Autodesk Fusion 360 part; units mm, degrees
(part 2 of 3)
pattern_linear "R-Pattern3" count 15 spacing 2.54 along (1, 0, 0) count 25 spacing 2.5396 along (0, 0, -1) of bodies 3 2 4 makes body 5 at (3.4863, 1, 63.5089) makes body 6 at (6.5468, 1, 62.4281) makes body 7 at (9.0868, 1, 63.5219) makes body 8 at (11.6268, 1, 63.5219) makes body 9 at (14.1668, 1, 63.5219) makes body 10 at (16.7068, 1, 63.5219) makes body 11 at (19.2468, 1, 63.5219) makes body 12 at (21.7868, 1, 63.5219) makes body 13 at (24.3268, 1, 63.5219) makes body 14 at (26.8668, 1, 63.5219) makes body 15 at (29.4068, 1, 63.5219) makes body 16 at (32.2529, 1, 63.2081) makes body 17 at (34.4868, 1, 63.5219) makes body 18 at (37.0268, 1, 63.5219) makes body 19 at (4.654, 0, 62.8955) makes body 20 at (7.194, 0, 62.8955) makes body 21 at (9.7359, 0, 62.9204) makes body 22 at (12.2759, 0, 62.9204) makes body 23 at (14.8159, 0, 62.9204) makes body 24 at (17.354, 0, 62.8955) makes body 25 at (19.894, 0, 62.8955) makes body 26 at (22.434, 0, 62.8955) makes body 27 at (24.974, 0, 62.8955) makes body 28 at (27.514, 0, 62.8955) makes body 29 at (30.054, 0, 62.8955) makes body 30 at (32.594, 0, 62.8955) makes body 31 at (35.134, 0, 62.8955) makes body 32 at (37.674, 0, 62.8955) makes body 33 at (4.654, 1.5, 62.8955) makes body 34 at (7.194, 1.5, 62.8955) makes body 35 at (9.7359, 1.5, 62.9204) makes body 36 at (12.2759, 1.5, 62.9204) makes body 37 at (14.8159, 1.5, 62.9204) makes body 38 at (17.354, 1.5, 62.8955) makes body 39 at (19.894, 1.5, 62.8955) makes body 40 at (22.434, 1.5, 62.8955) makes body 41 at (24.974, 1.5, 62.8955) makes body 42 at (27.514, 1.5, 62.8955) makes body 43 at (30.054, 1.5, 62.8955) makes body 44 at (32.594, 1.5, 62.8955) makes body 45 at (35.134, 1.5, 62.8955) makes body 46 at (37.674, 1.5, 62.8955) makes body 47 at (1.4668, 1, 60.9823) makes body 48 at (3.4863, 1, 60.9693) makes body 49 at (6.5468, 1, 59.8885) makes body 50 at (9.0868, 1, 60.9823) makes body 51 at (11.6268, 1, 60.9823) makes body 52 at (14.1668, 1, 60.9823) makes body 53 at (16.7068, 1, 60.9823) makes body 54 at (19.2468, 1, 60.9823) makes body 55 at (21.7868, 1, 60.9823) makes body 56 at (24.3268, 1, 60.9823) makes body 57 at (26.8668, 1, 60.9823) makes body 58 at (29.4068, 1, 60.9823) makes body 59 at (32.2529, 1, 60.6685) makes body 60 at (34.4868, 1, 60.9823) makes body 61 at (37.0268, 1, 60.9823) makes body 62 at (1.4668, 1, 58.4427) makes body 63 at (3.4863, 1, 58.4298) makes body 64 at (6.5468, 1, 57.3489) makes body 65 at (9.0868, 1, 58.4427) makes body 66 at (11.6268, 1, 58.4427) makes body 67 at (14.1668, 1, 58.4427) makes body 68 at (16.7068, 1, 58.4427) makes body 69 at (19.2468, 1, 58.4427) makes body 70 at (21.7868, 1, 58.4427) makes body 71 at (24.3268, 1, 58.4427) makes body 72 at (26.8668, 1, 58.4427) makes body 73 at (29.4068, 1, 58.4427) makes body 74 at (32.2529, 1, 58.1289) makes body 75 at (34.4868, 1, 58.4427) makes body 76 at (37.0268, 1, 58.4427) makes body 77 at (1.4668, 1, 55.9032) makes body 78 at (3.4863, 1, 55.8902) makes body 79 at (6.5468, 1, 54.8093) makes body 80 at (9.0868, 1, 55.9032) makes body 81 at (11.6268, 1, 55.9032) makes body 82 at (14.1668, 1, 55.9032) makes body 83 at (16.7068, 1, 55.9032) makes body 84 at (19.2468, 1, 55.9032) makes body 85 at (21.7868, 1, 55.9032) makes body 86 at (24.3268, 1, 55.9032) makes body 87 at (26.8668, 1, 55.9032) makes body 88 at (29.4068, 1, 55.9032) makes body 89 at (32.2529, 1, 55.5893) makes body 90 at (34.4868, 1, 55.9032) makes body 91 at (37.0268, 1, 55.9032) makes body 92 at (1.4668, 1, 53.3636) makes body 93 at (3.4863, 1, 53.3506) makes body 94 at (6.5468, 1, 52.2698) makes body 95 at (9.0868, 1, 53.3636) makes body 96 at (11.6268, 1, 53.3636) makes body 97 at (14.1668, 1, 53.3636) makes body 98 at (16.7068, 1, 53.3636) makes body 99 at (19.2468, 1, 53.3636) makes body 100 at (21.7868, 1, 53.3636) makes body 101 at (24.3268, 1, 53.3636) makes body 102 at (26.8668, 1, 53.3636) makes body 103 at (29.4068, 1, 53.3636) makes body 104 at (32.2529, 1, 53.0497) makes body 105 at (34.4868, 1, 53.3636) makes body 106 at (37.0268, 1, 53.3636) makes body 107 at (1.4668, 1, 50.824) makes body 108 at (3.4863, 1, 50.811) makes body 109 at (6.5468, 1, 49.7302) makes body 110 at (9.0868, 1, 50.824) makes body 111 at (11.6268, 1, 50.824) makes body 112 at (14.1668, 1, 50.824) makes body 113 at (16.7068, 1, 50.824) makes body 114 at (19.2468, 1, 50.824) makes body 115 at (21.7868, 1, 50.824) makes body 116 at (24.3268, 1, 50.824) makes body 117 at (26.8668, 1, 50.824) makes body 118 at (29.4068, 1, 50.824) makes body 119 at (32.2529, 1, 50.5101) makes body 120 at (34.4868, 1, 50.824) makes body 121 at (37.0268, 1, 50.824) makes body 122 at (1.4668, 1, 48.2844) makes body 123 at (3.4863, 1, 48.2714) makes body 124 at (6.5468, 1, 47.1906) makes body 125 at (9.0868, 1, 48.2844) makes body 126 at (11.6268, 1, 48.2844) makes body 127 at (14.1668, 1, 48.2844) makes body 128 at (16.7068, 1, 48.2844) makes body 129 at (19.2468, 1, 48.2844) makes body 130 at (21.7868, 1, 48.2844) makes body 131 at (24.3268, 1, 48.2844) makes body 132 at (26.8668, 1, 48.2844) makes body 133 at (29.4068, 1, 48.2844) makes body 134 at (32.2529, 1, 47.9706) makes body 135 at (34.4868, 1, 48.2844) makes body 136 at (37.0268, 1, 48.2844) makes body 137 at (1.4668, 1, 45.7448) makes body 138 at (3.4863, 1, 45.7318) makes body 139 at (6.5468, 1, 44.651) makes body 140 at (9.0868, 1, 45.7448) makes body 141 at (11.6268, 1, 45.7448) makes body 142 at (14.1668, 1, 45.7448) makes body 143 at (16.7068, 1, 45.7448) makes body 144 at (19.2468, 1, 45.7448) makes body 145 at (21.7868, 1, 45.7448) makes body 146 at (24.3268, 1, 45.7448) makes body 147 at (26.8668, 1, 45.7448) makes body 148 at (29.4068, 1, 45.7448) makes body 149 at (32.2529, 1, 45.431) makes body 150 at (34.4868, 1, 45.7448) makes body 151 at (37.0268, 1, 45.7448) makes body 152 at (1.4668, 1, 43.2052) makes body 153 at (3.4863, 1, 43.1923) makes body 154 at (6.5468, 1, 42.1114) makes body 155 at (9.0868, 1, 43.2052) makes body 156 at (11.6268, 1, 43.2052) makes body 157 at (14.1668, 1, 43.2052) makes body 158 at (16.7068, 1, 43.2052) makes body 159 at (19.2468, 1, 43.2052) makes body 160 at (21.7868, 1, 43.2052) makes body 161 at (24.3268, 1, 43.2052) makes body 162 at (26.8668, 1, 43.2052) makes body 163 at (29.4068, 1, 43.2052) makes body 164 at (32.2529, 1, 42.8914) makes body 165 at (34.4868, 1, 43.2052) makes body 166 at (37.0268, 1, 43.2052) makes body 167 at (1.4668, 1, 40.6657) makes body 168 at (3.4863, 1, 40.6527) makes body 169 at (6.5468, 1, 39.5718) makes body 170 at (9.0868, 1, 40.6657) makes body 171 at (11.6268, 1, 40.6657) makes body 172 at (14.1668, 1, 40.6657) makes body 173 at (16.7068, 1, 40.6657) makes body 174 at (19.2468, 1, 40.6657) makes body 175 at (21.7868, 1, 40.6657) makes body 176 at (24.3268, 1, 40.6657) makes body 177 at (26.8668, 1, 40.6657) makes body 178 at (29.4068, 1, 40.6657) makes body 179 at (32.2529, 1, 40.3518) makes body 180 at (34.4868, 1, 40.6657) makes body 181 at (37.0268, 1, 40.6657) makes body 182 at (1.4668, 1, 38.1261) makes body 183 at (3.4863, 1, 38.1131) makes body 184 at (6.5468, 1, 37.0323) makes body 185 at (9.0868, 1, 38.1261) makes body 186 at (11.6268, 1, 38.1261) makes body 187 at (14.1668, 1, 38.1261) makes body 188 at (16.7068, 1, 38.1261) makes body 189 at (19.2468, 1, 38.1261) makes body 190 at (21.7868, 1, 38.1261) makes body 191 at (24.3268, 1, 38.1261) makes body 192 at (26.8668, 1, 38.1261) makes body 193 at (29.4068, 1, 38.1261) makes body 194 at (32.2529, 1, 37.8122) makes body 195 at (34.4868, 1, 38.1261) makes body 196 at (37.0268, 1, 38.1261) makes body 197 at (1.4668, 1, 35.5865) makes body 198 at (3.4863, 1, 35.5735) makes body 199 at (6.5468, 1, 34.4927) makes body 200 at (9.0868, 1, 35.5865) makes body 201 at (11.6268, 1, 35.5865) makes body 202 at (14.1668, 1, 35.5865) makes body 203 at (16.7068, 1, 35.5865) makes body 204 at (19.2468, 1, 35.5865) makes body 205 at (21.7868, 1, 35.5865) makes body 206 at (24.3268, 1, 35.5865) makes body 207 at (26.8668, 1, 35.5865) makes body 208 at (29.4068, 1, 35.5865) makes body 209 at (32.2529, 1, 35.2726) makes body 210 at (34.4868, 1, 35.5865) makes body 211 at (37.0268, 1, 35.5865) makes body 212 at (1.4668, 1, 33.0469) makes body 213 at (3.4863, 1, 33.0339) makes body 214 at (6.8993, 0.5, 32.5299) makes body 215 at (9.0868, 1, 33.0469) makes body 216 at (11.6268, 1, 33.0469) makes body 217 at (14.1668, 1, 33.0469) makes body 218 at (16.7068, 1, 33.0469) makes body 219 at (19.2468, 1, 33.0469) makes body 220 at (21.7868, 1, 33.0469) makes body 221 at (24.3268, 1, 33.0469) makes body 222 at (26.8668, 1, 33.0469) makes body 223 at (29.4068, 1, 33.0469) makes body 224 at (32.2529, 1, 32.7331) makes body 225 at (34.4868, 1, 33.0469) makes body 226 at (37.0268, 1, 33.0469) makes body 227 at (1.8193, 1, 29.9305) makes body 228 at (4.3593, 1, 29.9305) makes body 229 at (6.8993, 1, 29.9305) makes body 230 at (9.4393, 1, 29.9305) makes body 231 at (11.9793, 1, 29.9305) makes body 232 at (14.5193, 1, 29.9305) makes body 233 at (17.0593, 1, 29.9305) makes body 234 at (19.5993, 1, 29.9305) makes body 235 at (22.1393, 1, 29.9305) makes body 236 at (24.6793, 1, 29.9305) makes body 237 at (27.2193, 1, 29.9305) makes body 238 at (29.7593, 1, 29.9305) makes body 239 at (32.2993, 1, 29.9305) makes body 240 at (34.5902, 1, 30.4476) makes body 241 at (37.1302, 1, 30.4476) makes body 242 at (1.8193, 1, 27.3909) makes body 243 at (4.3593, 1, 27.3909) makes body 244 at (6.8993, 1, 27.3909) makes body 245 at (9.4393, 1, 27.3909) makes body 246 at (11.9793, 1, 27.3909) makes body 247 at (14.5193, 1, 27.3909) makes body 248 at (17.0593, 1, 27.3909) makes body 249 at (19.5993, 1, 27.3909) makes body 250 at (22.1393, 1, 27.3909) makes body 251 at (24.6793, 1, 27.3909) makes body 252 at (27.2193, 1, 27.3909) makes body 253 at (29.7593, 1, 27.3909) makes body 254 at (32.2993, 1, 27.3909) makes body 255 at (34.5902, 1, 27.908) makes body 256 at (37.1302, 1, 27.908) makes body 257 at (1.8193, 1, 24.8513) makes body 258 at (4.3593, 1, 24.8513) makes body 259 at (6.8993, 1, 24.8513) makes body 260 at (9.4393, 1, 24.8513) makes body 261 at (11.9793, 1, 24.8513) makes body 262 at (14.5193, 1, 24.8513) makes body 263 at (17.0593, 1, 24.8513) makes body 264 at (19.5993, 1, 24.8513) makes body 265 at (22.1393, 1, 24.8513) makes body 266 at (24.6793, 1, 24.8513) makes body 267 at (27.2193, 1, 24.8513) makes body 268 at (29.7593, 1, 24.8513) makes body 269 at (32.2993, 1, 24.8513) makes body 270 at (34.5902, 1, 25.3684) makes body 271 at (37.1302, 1, 25.3684) makes body 272 at (1.8193, 1, 22.3118) makes body 273 at (4.3593, 1, 22.3118) makes body 274 at (6.8993, 1, 22.3118) makes body 275 at (9.4393, 1, 22.3118) makes body 276 at (11.9793, 1, 22.3118) makes body 277 at (14.5193, 1, 22.3118) makes body 278 at (17.0593, 1, 22.3118) makes body 279 at (19.5993, 1, 22.3118) makes body 280 at (22.1393, 1, 22.3118) makes body 281 at (24.6793, 1, 22.3118) makes body 282 at (27.2193, 1, 22.3118) makes body 283 at (29.7593, 1, 22.3118) makes body 284 at (32.2993, 1, 22.3118) makes body 285 at (34.5902, 1, 22.8288) makes body 286 at (37.1302, 1, 22.8288) makes body 287 at (1.8193, 1, 19.7722) makes body 288 at (4.3593, 1, 19.7722) makes body 289 at (6.8993, 1, 19.7722) makes body 290 at (9.4393, 1, 19.7722) makes body 291 at (11.9793, 1, 19.7722) makes body 292 at (14.5193, 1, 19.7722) makes body 293 at (17.0593, 1, 19.7722) makes body 294 at (19.5993, 1, 19.7722) makes body 295 at (22.1393, 1, 19.7722) makes body 296 at (24.6793, 1, 19.7722) makes body 297 at (27.2193, 1, 19.7722) makes body 298 at (29.7593, 1, 19.7722) makes body 299 at (32.2993, 1, 19.7722) makes body 300 at (34.5902, 1, 20.2892) makes body 301 at (37.1302, 1, 20.2892) makes body 302 at (1.8193, 1, 17.2326) makes body 303 at (4.3593, 1, 17.2326) makes body 304 at (6.8993, 1, 17.2326) makes body 305 at (9.4393, 1, 17.2326) makes body 306 at (11.9793, 1, 17.2326) makes body 307 at (14.5193, 1, 17.2326) makes body 308 at (17.0593, 1, 17.2326) makes body 309 at (19.5993, 1, 17.2326) makes body 310 at (22.1393, 1, 17.2326) makes body 311 at (24.6793, 1, 17.2326) makes body 312 at (27.2193, 1, 17.2326) makes body 313 at (29.7593, 1, 17.2326) makes body 314 at (32.2993, 1, 17.2326) makes body 315 at (34.5902, 1, 17.7497) makes body 316 at (37.1302, 1, 17.7497) makes body 317 at (0.7604, 1, 14.3372) makes body 318 at (4.157, 1, 15.1728) makes body 319 at (6.697, 1, 15.1728) makes body 320 at (9.237, 1, 15.1728) makes body 321 at (11.777, 1, 15.1728) makes body 322 at (14.317, 1, 15.1728) makes body 323 at (16.972, 1, 15.0358) makes body 324 at (19.512, 1, 15.0358) makes body 325 at (22.052, 1, 15.0358) makes body 326 at (24.592, 1, 15.0358) makes body 327 at (27.132, 1, 15.0358) makes body 328 at (29.672, 1, 15.0358) makes body 329 at (31.1731, 1, 15.0099) makes body 330 at (34.5902, 1, 15.2101) makes body 331 at (37.1302, 1, 15.2101) makes body 332 at (0.7604, 1, 11.7977) makes body 333 at (4.157, 1, 12.6332) makes body 334 at (6.697, 1, 12.6332) makes body 335 at (9.237, 1, 12.6332) makes body 336 at (11.777, 1, 12.6332) makes body 337 at (14.317, 1, 12.6332) makes body 338 at (16.972, 1, 12.4962) makes body 339 at (19.512, 1, 12.4962) makes body 340 at (22.052, 1, 12.4962) makes body 341 at (24.592, 1, 12.4962) makes body 342 at (27.132, 1, 12.4962) makes body 343 at (29.672, 1, 12.4962) makes body 344 at (31.1731, 1, 12.4703) makes body 345 at (34.5902, 1, 12.6705) makes body 346 at (37.1302, 1, 12.6705) makes body 347 at (0.7604, 1, 9.2581) makes body 348 at (4.157, 1, 10.0936) makes body 349 at (6.697, 1, 10.0936) makes body 350 at (9.237, 1, 10.0936) makes body 351 at (11.777, 1, 10.0936) makes body 352 at (14.317, 1, 10.0936) makes body 353 at (16.972, 1, 9.9566) makes body 354 at (19.512, 1, 9.9566) makes body 355 at (22.052, 1, 9.9566) makes body 356 at (24.592, 1, 9.9566) makes body 357 at (27.132, 1, 9.9566) makes body 358 at (29.672, 1, 9.9566) makes body 359 at (31.1731, 1, 9.9307) makes body 360 at (34.5902, 1, 10.1309) makes body 361 at (37.1302, 1, 10.1309) makes body 362 at (1.8193, 1, 7.0743) makes body 363 at (4.3593, 1, 7.0743) makes body 364 at (6.8993, 1, 7.0743) makes body 365 at (9.4393, 1, 7.0743) makes body 366 at (11.9793, 1, 7.0743) makes body 367 at (14.5193, 1, 7.0743) makes body 368 at (17.0593, 1, 7.0743) makes body 369 at (19.5993, 1, 7.0743) makes body 370 at (22.1393, 1, 7.0743) makes body 371 at (24.6793, 1, 7.0743) makes body 372 at (27.2193, 1, 7.0743) makes body 373 at (29.7593, 1, 7.0743) makes body 374 at (32.2529, 1, 7.3372) makes body 375 at (34.5902, 1, 7.5913) makes body 376 at (37.1302, 1, 7.5913) makes body 377 at (1.8193, 1, 4.5347) makes body 378 at (4.3593, 1, 4.5347) makes body 379 at (6.8993, 1, 4.5347) makes body 380 at (9.4393, 1, 4.5347) makes body 381 at (11.9793, 1, 4.5347) makes body 382 at (14.5193, 1, 4.5347) makes body 383 at (17.0593, 1, 4.5347) makes body 384 at (19.5993, 1, 4.5347) makes body 385 at (22.1393, 1, 4.5347) makes body 386 at (24.6793, 1, 4.5347) makes body 387 at (27.2193, 1, 4.5347) makes body 388 at (29.7593, 1, 4.5347) makes body 389 at (32.2529, 1, 4.7976) makes body 390 at (34.5902, 1, 5.0517) makes body 391 at (37.1302, 1, 5.0517) makes body 392 at (1.8193, 1, 1.9951) makes body 393 at (4.3593, 1, 1.9951) makes body 394 at (6.8993, 1, 1.9951) makes body 395 at (9.4393, 1, 1.9951) makes body 396 at (11.9793, 1, 1.9951) makes body 397 at (14.5193, 1, 1.9951) makes body 398 at (17.0593, 1, 1.9951) makes body 399 at (19.5993, 1, 1.9951) makes body 400 at (22.1393, 1, 1.9951) makes body 401 at (24.6793, 1, 1.9951) makes body 402 at (27.2193, 1, 1.9951) makes body 403 at (29.7593, 1, 1.9951) makes body 404 at (32.2529, 1, 2.2581) makes body 405 at (34.5902, 1, 2.5122) makes body 406 at (37.1302, 1, 2.5122) makes body 407 at (2.114, 0, 60.3559) makes body 408 at (4.654, 0, 60.3559) makes body 409 at (7.194, 0, 60.3559) makes body 410 at (9.7359, 0, 60.3808) makes body 411 at (12.2759, 0, 60.3808) makes body 412 at (14.8159, 0, 60.3808) makes body 413 at (17.354, 0, 60.3559) makes body 414 at (19.894, 0, 60.3559) makes body 415 at (22.434, 0, 60.3559) makes body 416 at (24.974, 0, 60.3559) makes body 417 at (27.514, 0, 60.3559) makes body 418 at (30.054, 0, 60.3559) makes body 419 at (32.594, 0, 60.3559) makes body 420 at (35.134, 0, 60.3559) makes body 421 at (37.674, 0, 60.3559) makes body 422 at (2.114, 0, 57.8163) makes body 423 at (4.654, 0, 57.8163) makes body 424 at (7.194, 0, 57.8163) makes body 425 at (9.7359, 0, 57.8412) makes body 426 at (12.2759, 0, 57.8412) makes body 427 at (14.8159, 0, 57.8412) makes body 428 at (17.354, 0, 57.8163) makes body 429 at (19.894, 0, 57.8163) makes body 430 at (22.434, 0, 57.8163) makes body 431 at (24.974, 0, 57.8163) makes body 432 at (27.514, 0, 57.8163) makes body 433 at (30.054, 0, 57.8163) makes body 434 at (32.594, 0, 57.8163) makes body 435 at (35.134, 0, 57.8163) makes body 436 at (37.674, 0, 57.8163) makes body 437 at (2.114, 0, 55.2768) makes body 438 at (4.654, 0, 55.2768) makes body 439 at (7.194, 0, 55.2768) makes body 440 at (9.7359, 0, 55.3016) makes body 441 at (12.2759, 0, 55.3016) makes body 442 at (14.8159, 0, 55.3016) makes body 443 at (17.354, 0, 55.2768) makes body 444 at (19.894, 0, 55.2768) makes body 445 at (22.434, 0, 55.2768) makes body 446 at (24.974, 0, 55.2768) makes body 447 at (27.514, 0, 55.2768) makes body 448 at (30.054, 0, 55.2768) makes body 449 at (32.594, 0, 55.2768) makes body 450 at (35.134, 0, 55.2768) makes body 451 at (37.674, 0, 55.2768) makes body 452 at (2.114, 0, 52.7372) makes body 453 at (4.654, 0, 52.7372) makes body 454 at (7.194, 0, 52.7372) makes body 455 at (9.7359, 0, 52.762) makes body 456 at (12.2759, 0, 52.762) makes body 457 at (14.8159, 0, 52.762) makes body 458 at (17.354, 0, 52.7372) makes body 459 at (19.894, 0, 52.7372) makes body 460 at (22.434, 0, 52.7372) makes body 461 at (24.974, 0, 52.7372) makes body 462 at (27.514, 0, 52.7372) makes body 463 at (30.054, 0, 52.7372) makes body 464 at (32.594, 0, 52.7372) makes body 465 at (35.134, 0, 52.7372) makes body 466 at (37.674, 0, 52.7372) makes body 467 at (2.114, 0, 50.1976) makes body 468 at (4.654, 0, 50.1976) makes body 469 at (7.194, 0, 50.1976) makes body 470 at (9.7359, 0, 50.2224) makes body 471 at (12.2759, 0, 50.2224) makes body 472 at (14.8159, 0, 50.2224) makes body 473 at (17.354, 0, 50.1976) makes body 474 at (19.894, 0, 50.1976) makes body 475 at (22.434, 0, 50.1976) makes body 476 at (24.974, 0, 50.1976) makes body 477 at (27.514, 0, 50.1976) makes body 478 at (30.054, 0, 50.1976) makes body 479 at (32.594, 0, 50.1976) makes body 480 at (35.134, 0, 50.1976) makes body 481 at (37.674, 0, 50.1976) makes body 482 at (2.114, 0, 47.658) makes body 483 at (4.654, 0, 47.658) makes body 484 at (7.194, 0, 47.658) makes body 485 at (9.734, 0, 47.658) makes body 486 at (12.274, 0, 47.658) makes body 487 at (14.814, 0, 47.658) makes body 488 at (17.354, 0, 47.658) makes body 489 at (19.894, 0, 47.658) makes body 490 at (22.434, 0, 47.658) makes body 491 at (24.974, 0, 47.658) makes body 492 at (27.514, 0, 47.658) makes body 493 at (30.054, 0, 47.658) makes body 494 at (32.594, 0, 47.658) makes body 495 at (35.134, 0, 47.658) makes body 496 at (37.674, 0, 47.658) makes body 497 at (2.114, 0, 45.1184) makes body 498 at (4.654, 0, 45.1184) makes body 499 at (7.194, 0, 45.1184) makes body 500 at (9.7359, 0, 45.1433) makes body 501 at (12.274, 0, 45.1184) makes body 502 at (14.814, 0, 45.1184) makes body 503 at (17.3559, 0, 45.1433) makes body 504 at (19.8959, 0, 45.1433) makes body 505 at (22.4359, 0, 45.1433) makes body 506 at (24.9759, 0, 45.1433) makes body 507 at (27.5159, 0, 45.1433) makes body 508 at (30.0559, 0, 45.1433) makes body 509 at (32.594, 0, 45.1184) makes body 510 at (35.1359, 0, 45.1433) makes body 511 at (37.6759, 0, 45.1433) makes body 512 at (2.114, 0, 42.5788) makes body 513 at (4.654, 0, 42.5788) makes body 514 at (7.194, 0, 42.5788) makes body 515 at (9.734, 0, 42.5788) makes body 516 at (12.274, 0, 42.5788) makes body 517 at (14.814, 0, 42.5788) makes body 518 at (17.354, 0, 42.5788) makes body 519 at (19.894, 0, 42.5788) makes body 520 at (22.434, 0, 42.5788) makes body 521 at (24.974, 0, 42.5788) makes body 522 at (27.514, 0, 42.5788) makes body 523 at (30.054, 0, 42.5788) makes body 524 at (32.594, 0, 42.5788) makes body 525 at (35.134, 0, 42.5788) makes body 526 at (37.674, 0, 42.5788) makes body 527 at (2.114, 0, 40.0393) makes body 528 at (4.654, 0, 40.0393) makes body 529 at (7.194, 0, 40.0393) makes body 530 at (9.7359, 0, 40.0641) makes body 531 at (12.274, 0, 40.0393) makes body 532 at (14.814, 0, 40.0393) makes body 533 at (17.3559, 0, 40.0641) makes body 534 at (19.8959, 0, 40.0641) makes body 535 at (22.4359, 0, 40.0641) makes body 536 at (24.9759, 0, 40.0641) makes body 537 at (27.5159, 0, 40.0641) makes body 538 at (30.0559, 0, 40.0641) makes body 539 at (32.594, 0, 40.0393) makes body 540 at (35.1359, 0, 40.0641) makes body 541 at (37.6759, 0, 40.0641) makes body 542 at (2.114, 0, 37.4997) makes body 543 at (4.654, 0, 37.4997) makes body 544 at (7.194, 0, 37.4997) makes body 545 at (9.734, 0, 37.4997) makes body 546 at (12.274, 0, 37.4997) makes body 547 at (14.814, 0, 37.4997) makes body 548 at (17.354, 0, 37.4997) makes body 549 at (19.894, 0, 37.4997) makes body 550 at (22.434, 0, 37.4997) makes body 551 at (24.974, 0, 37.4997) makes body 552 at (27.514, 0, 37.4997) makes body 553 at (30.054, 0, 37.4997) makes body 554 at (32.594, 0, 37.4997) makes body 555 at (35.134, 0, 37.4997) makes body 556 at (37.674, 0, 37.4997) makes body 557 at (2.114, 0, 34.9601) makes body 558 at (4.654, 0, 34.9601) makes body 559 at (7.194, 0, 34.9601) makes body 560 at (9.7359, 0, 34.9849) makes body 561 at (12.274, 0, 34.9601) makes body 562 at (14.814, 0, 34.9601) makes body 563 at (17.3559, 0, 34.9849) makes body 564 at (19.8959, 0, 34.9849) makes body 565 at (22.4359, 0, 34.9849) makes body 566 at (24.9759, 0, 34.9849) makes body 567 at (27.5159, 0, 34.9849) makes body 568 at (30.0559, 0, 34.9849) makes body 569 at (32.594, 0, 34.9601) makes body 570 at (35.1359, 0, 34.9849) makes body 571 at (37.6759, 0, 34.9849) makes body 572 at (2.114, 0, 32.4205) makes body 573 at (4.654, 0, 32.4205) makes body 574 at (7.194, 0, 32.4205) makes body 575 at (9.7359, 0, 32.4454) makes body 576 at (12.2759, 0, 32.4454) makes body 577 at (14.8159, 0, 32.4454) makes body 578 at (17.354, 0, 32.4205) makes body 579 at (19.894, 0, 32.4205) makes body 580 at (22.434, 0, 32.4205) makes body 581 at (24.974, 0, 32.4205) makes body 582 at (27.514, 0, 32.4205) makes body 583 at (30.054, 0, 32.4205) makes body 584 at (32.594, 0, 32.4205) makes body 585 at (35.134, 0, 32.4205) makes body 586 at (37.674, 0, 32.4205) makes body 587 at (2.114, 0, 29.8809) makes body 588 at (4.654, 0, 29.8809) makes body 589 at (7.194, 0, 29.8809) makes body 590 at (9.7359, 0, 29.9058) makes body 591 at (10.4841, 0, 29.9058) makes body 592 at (13.0241, 0, 29.9058) makes body 593 at (17.354, 0, 29.8809) makes body 594 at (18.1041, 0, 29.9058) makes body 595 at (20.6441, 0, 29.9058) makes body 596 at (23.1841, 0, 29.9058) makes body 597 at (25.7241, 0, 29.9058) makes body 598 at (28.2641, 0, 29.9058) makes body 599 at (32.1006, 0, 29.1572) makes body 600 at (33.4565, 0, 29.5225) makes body 601 at (35.9965, 0, 29.5225) makes body 602 at (2.114, 0, 27.3413) makes body 603 at (4.654, 0, 27.3413) makes body 604 at (7.194, 0, 27.3413) makes body 605 at (9.7359, 0, 27.3662) makes body 606 at (10.4841, 0, 27.3662) makes body 607 at (13.0241, 0, 27.3662) makes body 608 at (17.354, 0, 27.3413) makes body 609 at (18.1041, 0, 27.3662) makes body 610 at (20.6441, 0, 27.3662) makes body 611 at (23.1841, 0, 27.3662) makes body 612 at (25.7241, 0, 27.3662) makes body 613 at (28.2641, 0, 27.3662) makes body 614 at (32.1006, 0, 26.6176) makes body 615 at (33.4565, 0, 26.9829) makes body 616 at (35.9965, 0, 26.9829) makes body 617 at (2.114, 0, 24.8018) makes body 618 at (4.654, 0, 24.8018) makes body 619 at (7.194, 0, 24.8018) makes body 620 at (9.7359, 0, 24.8266) makes body 621 at (10.4841, 0, 24.8266) makes body 622 at (13.0241, 0, 24.8266) makes body 623 at (17.354, 0, 24.8018) makes body 624 at (18.1041, 0, 24.8266) makes body 625 at (20.6441, 0, 24.8266) makes body 626 at (23.1841, 0, 24.8266) makes body 627 at (25.7241, 0, 24.8266) makes body 628 at (28.2641, 0, 24.8266) makes body 629 at (32.1006, 0, 24.078) makes body 630 at (33.4565, 0, 24.4433) makes body 631 at (35.9965, 0, 24.4433) makes body 632 at (2.114, 0, 22.2622) makes body 633 at (4.654, 0, 22.2622) makes body 634 at (7.194, 0, 22.2622) makes body 635 at (9.7359, 0, 22.287) makes body 636 at (10.4841, 0, 22.287) makes body 637 at (13.0241, 0, 22.287) makes body 638 at (17.354, 0, 22.2622) makes body 639 at (18.1041, 0, 22.287) makes body 640 at (20.6441, 0, 22.287) makes body 641 at (23.1841, 0, 22.287) makes body 642 at (25.7241, 0, 22.287) makes body 643 at (28.2641, 0, 22.287) makes body 644 at (32.1006, 0, 21.5385) makes body 645 at (33.4565, 0, 21.9037) makes body 646 at (35.9965, 0, 21.9037) makes body 647 at (2.114, 0, 19.7226) makes body 648 at (4.654, 0, 19.7226) makes body 649 at (7.194, 0, 19.7226) makes body 650 at (9.7359, 0, 19.7474) makes body 651 at (10.4841, 0, 19.7474) makes body 652 at (13.0241, 0, 19.7474) makes body 653 at (17.354, 0, 19.7226) makes body 654 at (18.1041, 0, 19.7474) makes body 655 at (20.6441, 0, 19.7474) makes body 656 at (23.1841, 0, 19.7474) makes body 657 at (25.7241, 0, 19.7474) makes body 658 at (28.2641, 0, 19.7474) makes body 659 at (32.1006, 0, 18.9989) makes body 660 at (33.4565, 0, 19.3641) makes body 661 at (35.9965, 0, 19.3641) makes body 662 at (2.114, 0, 17.183) makes body 663 at (4.654, 0, 17.183) makes body 664 at (7.194, 0, 17.183) makes body 665 at (9.7359, 0, 17.2079) makes body 666 at (10.4841, 0, 17.2079) makes body 667 at (13.0241, 0, 17.2079) makes body 668 at (17.354, 0, 17.183) makes body 669 at (18.1041, 0, 17.2079) makes body 670 at (20.6441, 0, 17.2079) makes body 671 at (23.1841, 0, 17.2079) makes body 672 at (25.7241, 0, 17.2079) makes body 673 at (28.2641, 0, 17.2079) makes body 674 at (32.1006, 0, 16.4593) makes body 675 at (33.4565, 0, 16.8245) makes body 676 at (35.9965, 0, 16.8245) makes body 677 at (2.114, 0, 14.6434) makes body 678 at (4.654, 0, 14.6434) makes body 679 at (7.194, 0, 14.6434) makes body 680 at (9.7359, 0, 14.6683) makes body 681 at (12.2759, 0, 14.6683) makes body 682 at (14.8159, 0, 14.6683) makes body 683 at (17.2435, 0, 15.1609) makes body 684 at (19.7835, 0, 15.1609) makes body 685 at (22.3235, 0, 15.1609) makes body 686 at (24.8635, 0, 15.1609) makes body 687 at (27.4035, 0, 15.1609) makes body 688 at (30.054, 0, 14.6434) makes body 689 at (32.1006, 0, 13.9197) makes body 690 at (33.4565, 0, 14.285) makes body 691 at (35.9965, 0, 14.285) makes body 692 at (2.114, 0, 12.1038) makes body 693 at (4.654, 0, 12.1038) makes body 694 at (7.194, 0, 12.1038) makes body 695 at (9.7359, 0, 12.1287) makes body 696 at (12.2759, 0, 12.1287) makes body 697 at (14.8159, 0, 12.1287) makes body 698 at (17.2435, 0, 12.6213) makes body 699 at (19.7835, 0, 12.6213) makes body 700 at (22.3235, 0, 12.6213) makes body 701 at (24.8635, 0, 12.6213) makes body 702 at (27.4035, 0, 12.6213) makes body 703 at (30.054, 0, 12.1038) makes body 704 at (32.1006, 0, 11.3801) makes body 705 at (33.4565, 0, 11.7454) makes body 706 at (35.9965, 0, 11.7454) makes body 707 at (2.114, 0, 9.5643) makes body 708 at (4.654, 0, 9.5643) makes body 709 at (7.194, 0, 9.5643) makes body 710 at (9.7359, 0, 9.5891) makes body 711 at (12.2759, 0, 9.5891) makes body 712 at (14.8159, 0, 9.5891) makes body 713 at (17.2435, 0, 10.0817) makes body 714 at (19.7835, 0, 10.0817) makes body 715 at (22.3235, 0, 10.0817) makes body 716 at (24.8635, 0, 10.0817) makes body 717 at (27.4035, 0, 10.0817) makes body 718 at (30.054, 0, 9.5643) makes body 719 at (32.1006, 0, 8.8405) makes body 720 at (33.4565, 0, 9.2058) makes body 721 at (35.9965, 0, 9.2058) makes body 722 at (2.114, 0, 7.0247) makes body 723 at (4.654, 0, 7.0247) makes body 724 at (7.194, 0, 7.0247) makes body 725 at (9.7359, 0, 7.0495) makes body 726 at (12.2759, 0, 7.0495) makes body 727 at (14.8159, 0, 7.0495) makes body 728 at (17.354, 0, 7.0247) makes body 729 at (19.894, 0, 7.0247) makes body 730 at (22.434, 0, 7.0247) makes body 731 at (24.974, 0, 7.0247) makes body 732 at (27.514, 0, 7.0247) makes body 733 at (30.054, 0, 7.0247) makes body 734 at (32.1006, 0, 6.301) makes body 735 at (35.0235, 0, 6.6662) makes body 736 at (37.5635, 0, 6.6662) makes body 737 at (2.114, 0, 4.4851) makes body 738 at (4.654, 0, 4.4851) makes body 739 at (7.194, 0, 4.4851) makes body 740 at (9.7359, 0, 4.5099) makes body 741 at (12.2759, 0, 4.5099) makes body 742 at (14.8159, 0, 4.5099) makes body 743 at (17.354, 0, 4.4851) makes body 744 at (19.894, 0, 4.4851) makes body 745 at (22.434, 0, 4.4851) makes body 746 at (24.974, 0, 4.4851) makes body 747 at (27.514, 0, 4.4851) makes body 748 at (30.054, 0, 4.4851) makes body 749 at (32.1006, 0, 3.7614) makes body 750 at (33.4565, 0, 4.1266) makes body 751 at (35.9965, 0, 4.1266) makes body 752 at (2.114, 0, 1.9455) makes body 753 at (4.654, 0, 1.9455) makes body 754 at (7.194, 0, 1.9455) makes body 755 at (9.7359, 0, 1.9704) makes body 756 at (12.2759, 0, 1.9704) makes body 757 at (14.8159, 0, 1.9704) makes body 758 at (17.354, 0, 1.9455) makes body 759 at (19.894, 0, 1.9455) makes body 760 at (22.434, 0, 1.9455) makes body 761 at (24.974, 0, 1.9455) makes body 762 at (27.514, 0, 1.9455) makes body 763 at (30.054, 0, 1.9455) makes body 764 at (32.1006, 0, 1.2218) makes body 765 at (33.4565, 0, 1.587) makes body 766 at (35.9965, 0, 1.587) makes body 767 at (2.114, 1.5, 60.3559) makes body 768 at (4.654, 1.5, 60.3559) makes body 769 at (7.194, 1.5, 60.3559) makes body 770 at (9.7359, 1.5, 60.3808) makes body 771 at (12.2759, 1.5, 60.3808) makes body 772 at (14.8159, 1.5, 60.3808) makes body 773 at (17.354, 1.5, 60.3559) makes body 774 at (19.894, 1.5, 60.3559) makes body 775 at (22.434, 1.5, 60.3559) makes body 776 at (24.974, 1.5, 60.3559) makes body 777 at (27.514, 1.5, 60.3559) makes body 778 at (30.054, 1.5, 60.3559) makes body 779 at (32.594, 1.5, 60.3559) makes body 780 at (35.134, 1.5, 60.3559) makes body 781 at (37.674, 1.5, 60.3559) makes body 782 at (2.114, 1.5, 57.8163) makes body 783 at (4.654, 1.5, 57.8163) makes body 784 at (7.194, 1.5, 57.8163) makes body 785 at (9.7359, 1.5, 57.8412) makes body 786 at (12.2759, 1.5, 57.8412) makes body 787 at (14.8159, 1.5, 57.8412) makes body 788 at (17.354, 1.5, 57.8163) makes body 789 at (19.894, 1.5, 57.8163) makes body 790 at (22.434, 1.5, 57.8163) makes body 791 at (24.974, 1.5, 57.8163) makes body 792 at (27.514, 1.5, 57.8163) makes body 793 at (30.054, 1.5, 57.8163) makes body 794 at (32.594, 1.5, 57.8163) makes body 795 at (35.134, 1.5, 57.8163) makes body 796 at (37.674, 1.5, 57.8163) makes body 797 at (2.114, 1.5, 55.2768) makes body 798 at (4.654, 1.5, 55.2768) makes body 799 at (7.194, 1.5, 55.2768) makes body 800 at (9.7359, 1.5, 55.3016) makes body 801 at (12.2759, 1.5, 55.3016) makes body 802 at (14.8159, 1.5, 55.3016) makes body 803 at (17.354, 1.5, 55.2768) makes body 804 at (19.894, 1.5, 55.2768) makes body 805 at (22.434, 1.5, 55.2768) makes body 806 at (24.974, 1.5, 55.2768) makes body 807 at (27.514, 1.5, 55.2768) makes body 808 at (30.054, 1.5, 55.2768) makes body 809 at (32.594, 1.5, 55.2768) makes body 810 at (35.134, 1.5, 55.2768) makes body 811 at (37.674, 1.5, 55.2768) makes body 812 at (2.114, 1.5, 52.7372) makes body 813 at (4.654, 1.5, 52.7372) makes body 814 at (7.194, 1.5, 52.7372) makes body 815 at (9.7359, 1.5, 52.762) makes body 816 at (12.2759, 1.5, 52.762) makes body 817 at (14.8159, 1.5, 52.762) makes body 818 at (17.354, 1.5, 52.7372) makes body 819 at (19.894, 1.5, 52.7372) makes body 820 at (22.434, 1.5, 52.7372) makes body 821 at (24.974, 1.5, 52.7372) makes body 822 at (27.514, 1.5, 52.7372) makes body 823 at (30.054, 1.5, 52.7372) makes body 824 at (32.594, 1.5, 52.7372) makes body 825 at (35.134, 1.5, 52.7372) makes body 826 at (37.674, 1.5, 52.7372) makes body 827 at (2.114, 1.5, 50.1976) makes body 828 at (4.654, 1.5, 50.1976) makes body 829 at (7.194, 1.5, 50.1976) makes body 830 at (9.7359, 1.5, 50.2224) makes body 831 at (12.2759, 1.5, 50.2224) makes body 832 at (14.8159, 1.5, 50.2224) makes body 833 at (17.354, 1.5, 50.1976) makes body 834 at (19.894, 1.5, 50.1976) makes body 835 at (22.434, 1.5, 50.1976) makes body 836 at (24.974, 1.5, 50.1976) makes body 837 at (27.514, 1.5, 50.1976) makes body 838 at (30.054, 1.5, 50.1976) makes body 839 at (32.594, 1.5, 50.1976) makes body 840 at (35.134, 1.5, 50.1976) makes body 841 at (37.674, 1.5, 50.1976) makes body 842 at (2.114, 1.5, 47.658) makes body 843 at (4.654, 1.5, 47.658) makes body 844 at (7.194, 1.5, 47.658) makes body 845 at (9.734, 1.5, 47.658) makes body 846 at (12.274, 1.5, 47.658) makes body 847 at (14.814, 1.5, 47.658) makes body 848 at (17.354, 1.5, 47.658) makes body 849 at (19.894, 1.5, 47.658) makes body 850 at (22.434, 1.5, 47.658) makes body 851 at (24.974, 1.5, 47.658) makes body 852 at (27.514, 1.5, 47.658) makes body 853 at (30.054, 1.5, 47.658) makes body 854 at (32.594, 1.5, 47.658) makes body 855 at (35.134, 1.5, 47.658) makes body 856 at (37.674, 1.5, 47.658) makes body 857 at (2.114, 1.5, 45.1184) makes body 858 at (4.654, 1.5, 45.1184) makes body 859 at (7.194, 1.5, 45.1184) makes body 860 at (9.7359, 1.5, 45.1433) makes body 861 at (12.274, 1.5, 45.1184) makes body 862 at (14.814, 1.5, 45.1184) makes body 863 at (17.3559, 1.5, 45.1433) makes body 864 at (19.8959, 1.5, 45.1433) makes body 865 at (22.4359, 1.5, 45.1433) makes body 866 at (24.9759, 1.5, 45.1433) makes body 867 at (27.5159, 1.5, 45.1433) makes body 868 at (30.0559, 1.5, 45.1433) makes body 869 at (32.594, 1.5, 45.1184) makes body 870 at (35.1359, 1.5, 45.1433) makes body 871 at (37.6759, 1.5, 45.1433) makes body 872 at (2.114, 1.5, 42.5788) makes body 873 at (4.654, 1.5, 42.5788) makes body 874 at (7.194, 1.5, 42.5788) makes body 875 at (9.734, 1.5, 42.5788) makes body 876 at (12.274, 1.5, 42.5788) makes body 877 at (14.814, 1.5, 42.5788) makes body 878 at (17.354, 1.5, 42.5788) makes body 879 at (19.894, 1.5, 42.5788) makes body 880 at (22.434, 1.5, 42.5788) makes body 881 at (24.974, 1.5, 42.5788) makes body 882 at (27.514, 1.5, 42.5788) makes body 883 at (30.054, 1.5, 42.5788) makes body 884 at (32.594, 1.5, 42.5788) makes body 885 at (35.134, 1.5, 42.5788) makes body 886 at (37.674, 1.5, 42.5788) makes body 887 at (2.114, 1.5, 40.0393) makes body 888 at (4.654, 1.5, 40.0393) makes body 889 at (7.194, 1.5, 40.0393) makes body 890 at (9.7359, 1.5, 40.0641) makes body 891 at (12.274, 1.5, 40.0393) makes body 892 at (14.814, 1.5, 40.0393) makes body 893 at (17.3559, 1.5, 40.0641) makes body 894 at (19.8959, 1.5, 40.0641) makes body 895 at (22.4359, 1.5, 40.0641) makes body 896 at (24.9759, 1.5, 40.0641) makes body 897 at (27.5159, 1.5, 40.0641) makes body 898 at (30.0559, 1.5, 40.0641) makes body 899 at (32.594, 1.5, 40.0393) makes body 900 at (35.1359, 1.5, 40.0641) makes body 901 at (37.6759, 1.5, 40.0641) makes body 902 at (2.114, 1.5, 37.4997) makes body 903 at (4.654, 1.5, 37.4997) makes body 904 at (7.194, 1.5, 37.4997) makes body 905 at (9.734, 1.5, 37.4997) makes body 906 at (12.274, 1.5, 37.4997) makes body 907 at (14.814, 1.5, 37.4997) makes body 908 at (17.354, 1.5, 37.4997) makes body 909 at (19.894, 1.5, 37.4997) makes body 910 at (22.434, 1.5, 37.4997) makes body 911 at (24.974, 1.5, 37.4997) makes body 912 at (27.514, 1.5, 37.4997) makes body 913 at (30.054, 1.5, 37.4997) makes body 914 at (32.594, 1.5, 37.4997) makes body 915 at (35.134, 1.5, 37.4997) makes body 916 at (37.674, 1.5, 37.4997) makes body 917 at (2.114, 1.5, 34.9601) makes body 918 at (4.654, 1.5, 34.9601) makes body 919 at (7.194, 1.5, 34.9601) makes body 920 at (9.7359, 1.5, 34.9849) makes body 921 at (12.274, 1.5, 34.9601) makes body 922 at (14.814, 1.5, 34.9601) makes body 923 at (17.3559, 1.5, 34.9849) makes body 924 at (19.8959, 1.5, 34.9849) makes body 925 at (22.4359, 1.5, 34.9849) makes body 926 at (24.9759, 1.5, 34.9849) makes body 927 at (27.5159, 1.5, 34.9849) makes body 928 at (30.0559, 1.5, 34.9849) makes body 929 at (32.594, 1.5, 34.9601) makes body 930 at (35.1359, 1.5, 34.9849) makes body 931 at (37.6759, 1.5, 34.9849) makes body 932 at (2.114, 1.5, 32.4205) makes body 933 at (4.654, 1.5, 32.4205) makes body 934 at (7.194, 1.5, 32.4205) makes body 935 at (9.7359, 1.5, 32.4454) makes body 936 at (12.2759, 1.5, 32.4454) makes body 937 at (14.8159, 1.5, 32.4454) makes body 938 at (17.354, 1.5, 32.4205) makes body 939 at (19.894, 1.5, 32.4205) makes body 940 at (22.434, 1.5, 32.4205) makes body 941 at (24.974, 1.5, 32.4205) makes body 942 at (27.514, 1.5, 32.4205) makes body 943 at (30.054, 1.5, 32.4205) makes body 944 at (32.594, 1.5, 32.4205) makes body 945 at (35.134, 1.5, 32.4205) makes body 946 at (37.674, 1.5, 32.4205) makes body 947 at (2.114, 1.5, 29.8809) makes body 948 at (4.654, 1.5, 29.8809) makes body 949 at (7.194, 1.5, 29.8809) makes body 950 at (9.7359, 1.5, 29.9058) makes body 951 at (10.4841, 1.5, 29.9058) makes body 952 at (13.0241, 1.5, 29.9058) makes body 953 at (17.354, 1.5, 29.8809) makes body 954 at (18.1041, 1.5, 29.9058) makes body 955 at (20.6441, 1.5, 29.9058) makes body 956 at (23.1841, 1.5, 29.9058) makes body 957 at (25.7241, 1.5, 29.9058) makes body 958 at (28.2641, 1.5, 29.9058) makes body 959 at (32.1006, 1.5, 29.1572) makes body 960 at (33.4565, 1.5, 29.5225) makes body 961 at (35.9965, 1.5, 29.5225) makes body 962 at (2.114, 1.5, 27.3413) makes body 963 at (4.654, 1.5, 27.3413) makes body 964 at (7.194, 1.5, 27.3413) makes body 965 at (9.7359, 1.5, 27.3662) makes body 966 at (10.4841, 1.5, 27.3662) makes body 967 at (13.0241, 1.5, 27.3662) makes body 968 at (17.354, 1.5, 27.3413) makes body 969 at (18.1041, 1.5, 27.3662) makes body 970 at (20.6441, 1.5, 27.3662) makes body 971 at (23.1841, 1.5, 27.3662) makes body 972 at (25.7241, 1.5, 27.3662) makes body 973 at (28.2641, 1.5, 27.3662) makes body 974 at (32.1006, 1.5, 26.6176) makes body 975 at (33.4565, 1.5, 26.9829) makes body 976 at (35.9965, 1.5, 26.9829) makes body 977 at (2.114, 1.5, 24.8018) makes body 978 at (4.654, 1.5, 24.8018) makes body 979 at (7.194, 1.5, 24.8018) makes body 980 at (9.7359, 1.5, 24.8266) makes body 981 at (10.4841, 1.5, 24.8266) makes body 982 at (13.0241, 1.5, 24.8266) makes body 983 at (17.354, 1.5, 24.8018) makes body 984 at (18.1041, 1.5, 24.8266) makes body 985 at (20.6441, 1.5, 24.8266) makes body 986 at (23.1841, 1.5, 24.8266) makes body 987 at (25.7241, 1.5, 24.8266) makes body 988 at (28.2641, 1.5, 24.8266) makes body 989 at (32.1006, 1.5, 24.078) makes body 990 at (33.4565, 1.5, 24.4433) makes body 991 at (35.9965, 1.5, 24.4433) makes body 992 at (2.114, 1.5, 22.2622) makes body 993 at (4.654, 1.5, 22.2622) makes body 994 at (7.194, 1.5, 22.2622) makes body 995 at (9.7359, 1.5, 22.287) makes body 996 at (10.4841, 1.5, 22.287) makes body 997 at (13.0241, 1.5, 22.287) makes body 998 at (17.354, 1.5, 22.2622) makes body 999 at (18.1041, 1.5, 22.287) makes body 1000 at (20.6441, 1.5, 22.287) makes body 1001 at (23.1841, 1.5, 22.287) makes body 1002 at (25.7241, 1.5, 22.287) makes body 1003 at (28.2641, 1.5, 22.287) makes body 1004 at (32.1006, 1.5, 21.5385) makes body 1005 at (33.4565, 1.5, 21.9037) makes body 1006 at (35.9965, 1.5, 21.9037) makes body 1007 at (2.114, 1.5, 19.7226) makes body 1008 at (4.654, 1.5, 19.7226) makes body 1009 at (7.194, 1.5, 19.7226) makes body 1010 at (9.7359, 1.5, 19.7474) makes body 1011 at (10.4841, 1.5, 19.7474) makes body 1012 at (13.0241, 1.5, 19.7474) makes body 1013 at (17.354, 1.5, 19.7226) makes body 1014 at (18.1041, 1.5, 19.7474) makes body 1015 at (20.6441, 1.5, 19.7474) makes body 1016 at (23.1841, 1.5, 19.7474) makes body 1017 at (25.7241, 1.5, 19.7474) makes body 1018 at (28.2641, 1.5, 19.7474) makes body 1019 at (32.1006, 1.5, 18.9989) makes body 1020 at (33.4565, 1.5, 19.3641) makes body 1021 at (35.9965, 1.5, 19.3641) makes body 1022 at (2.114, 1.5, 17.183) makes body 1023 at (4.654, 1.5, 17.183) makes body 1024 at (7.194, 1.5, 17.183) makes body 1025 at (9.7359, 1.5, 17.2079) makes body 1026 at (10.4841, 1.5, 17.2079) makes body 1027 at (13.0241, 1.5, 17.2079) makes body 1028 at (17.354, 1.5, 17.183) makes body 1029 at (18.1041, 1.5, 17.2079) makes body 1030 at (20.6441, 1.5, 17.2079) makes body 1031 at (23.1841, 1.5, 17.2079) makes body 1032 at (25.7241, 1.5, 17.2079) makes body 1033 at (28.2641, 1.5, 17.2079) makes body 1034 at (32.1006, 1.5, 16.4593) makes body 1035 at (33.4565, 1.5, 16.8245) makes body 1036 at (35.9965, 1.5, 16.8245) makes body 1037 at (2.114, 1.5, 14.6434) makes body 1038 at (4.654, 1.5, 14.6434) makes body 1039 at (7.194, 1.5, 14.6434) makes body 1040 at (9.7359, 1.5, 14.6683) makes body 1041 at (12.2759, 1.5, 14.6683) makes body 1042 at (14.8159, 1.5, 14.6683) makes body 1043 at (17.2435, 1.5, 15.1609) makes body 1044 at (19.7835, 1.5, 15.1609) makes body 1045 at (22.3235, 1.5, 15.1609) makes body 1046 at (24.8635, 1.5, 15.1609) makes body 1047 at (27.4035, 1.5, 15.1609) makes body 1048 at (30.054, 1.5, 14.6434) makes body 1049 at (32.1006, 1.5, 13.9197) makes body 1050 at (33.4565, 1.5, 14.285) makes body 1051 at (35.9965, 1.5, 14.285) makes body 1052 at (2.114, 1.5, 12.1038) makes body 1053 at (4.654, 1.5, 12.1038) makes body 1054 at (7.194, 1.5, 12.1038) makes body 1055 at (9.7359, 1.5, 12.1287) makes body 1056 at (12.2759, 1.5, 12.1287) makes body 1057 at (14.8159, 1.5, 12.1287) makes body 1058 at (17.2435, 1.5, 12.6213) makes body 1059 at (19.7835, 1.5, 12.6213) makes body 1060 at (22.3235, 1.5, 12.6213) makes body 1061 at (24.8635, 1.5, 12.6213) makes body 1062 at (27.4035, 1.5, 12.6213) makes body 1063 at (30.054, 1.5, 12.1038) makes body 1064 at (32.1006, 1.5, 11.3801) makes body 1065 at (33.4565, 1.5, 11.7454) makes body 1066 at (35.9965, 1.5, 11.7454) makes body 1067 at (2.114, 1.5, 9.5643) makes body 1068 at (4.654, 1.5, 9.5643) makes body 1069 at (7.194, 1.5, 9.5643) makes body 1070 at (9.7359, 1.5, 9.5891) makes body 1071 at (12.2759, 1.5, 9.5891) makes body 1072 at (14.8159, 1.5, 9.5891) makes body 1073 at (17.2435, 1.5, 10.0817) makes body 1074 at (19.7835, 1.5, 10.0817) makes body 1075 at (22.3235, 1.5, 10.0817) makes body 1076 at (24.8635, 1.5, 10.0817) makes body 1077 at (27.4035, 1.5, 10.0817) makes body 1078 at (30.054, 1.5, 9.5643) makes body 1079 at (32.1006, 1.5, 8.8405) makes body 1080 at (33.4565, 1.5, 9.2058) makes body 1081 at (35.9965, 1.5, 9.2058) makes body 1082 at (2.114, 1.5, 7.0247) makes body 1083 at (4.654, 1.5, 7.0247) makes body 1084 at (7.194, 1.5, 7.0247) makes body 1085 at (9.7359, 1.5, 7.0495) makes body 1086 at (12.2759, 1.5, 7.0495) makes body 1087 at (14.8159, 1.5, 7.0495) makes body 1088 at (17.354, 1.5, 7.0247) makes body 1089 at (19.894, 1.5, 7.0247) makes body 1090 at (22.434, 1.5, 7.0247) makes body 1091 at (24.974, 1.5, 7.0247) makes body 1092 at (27.514, 1.5, 7.0247) makes body 1093 at (30.054, 1.5, 7.0247) makes body 1094 at (32.1006, 1.5, 6.301) makes body 1095 at (35.0235, 1.5, 6.6662) makes body 1096 at (37.5635, 1.5, 6.6662) makes body 1097 at (2.114, 1.5, 4.4851) makes body 1098 at (4.654, 1.5, 4.4851) makes body 1099 at (7.194, 1.5, 4.4851) makes body 1100 at (9.7359, 1.5, 4.5099) makes body 1101 at (12.2759, 1.5, 4.5099) makes body 1102 at (14.8159, 1.5, 4.5099) makes body 1103 at (17.354, 1.5, 4.4851) makes body 1104 at (19.894, 1.5, 4.4851) makes body 1105 at (22.434, 1.5, 4.4851) makes body 1106 at (24.974, 1.5, 4.4851) makes body 1107 at (27.514, 1.5, 4.4851) makes body 1108 at (30.054, 1.5, 4.4851) makes body 1109 at (32.1006, 1.5, 3.7614) makes body 1110 at (33.4565, 1.5, 4.1266) makes body 1111 at (35.9965, 1.5, 4.1266) makes body 1112 at (2.114, 1.5, 1.9455) makes body 1113 at (4.654, 1.5, 1.9455) makes body 1114 at (7.194, 1.5, 1.9455) makes body 1115 at (9.7359, 1.5, 1.9704) makes body 1116 at (12.2759, 1.5, 1.9704) makes body 1117 at (14.8159, 1.5, 1.9704) makes body 1118 at (17.354, 1.5, 1.9455) makes body 1119 at (19.894, 1.5, 1.9455) makes body 1120 at (22.434, 1.5, 1.9455) makes body 1121 at (24.974, 1.5, 1.9455) makes body 1122 at (27.514, 1.5, 1.9455) makes body 1123 at (30.054, 1.5, 1.9455) makes body 1124 at (32.1006, 1.5, 1.2218) makes body 1125 at (33.4565, 1.5, 1.587) makes body 1126 at (35.9965, 1.5, 1.587)
equation "d12 = 0.72 mm + 0.5 mm"